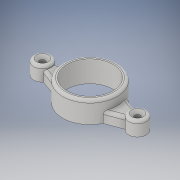
# Autodesk Inventor part: Counter_Support
Saved by Autodesk Inventor 2017 (Build 210142000, 142)
## iProperties
Created: 2019-12-30
Part Number: Counter_Support
Material: Generic
Document SubType Name: Modeling
Designer: Christian
Density: 1 g/cm^3
Appearance: Default
Author: Christian
Autodesk Inventor part; units mm, degrees
ref_plane "YZ Plane" through (0, 0, 0) normal (1, 0, 0) x (0, 1, 0)
ref_plane "XZ Plane" through (0, 0, 0) normal (0, 1, 0) x (-1, 0, 0)
ref_plane "XY Plane" through (0, 0, 0) normal (0, 0, 1) x (1, 0, 0)
sketch "Tube_Core_Skt" plane through (0, 0, 0) normal (0, 0, 1) x (1, 0, 0)
  circle A0 centre (0, 0) radius 16.025
  circle A1 centre (0, 0) radius 19.025
  dimension "d2" = 3
  dimension "d3" = 32.05
  constraints: 2 centre point, 2 coincident
  measures "d2" radial gap between concentric circles of A1 A0
  measures "d3" diameter of A0
extrude "Tube_Core" add sketch "Tube_Core_Skt" along normal blind 15
sketch "Screw_Core_Skt" plane through (0, 0, 0) normal (0, 1, 0) x (-1, 0, 0)
  line L0 (-19.025, 0) -> (-19.025, 15) projected
  line L1 (19.025, 15) -> (-19.025, 15) projected
  line L2 (19.025, 0) -> (19.025, 15) projected
  line L3 (-19.025, 0) -> (19.025, 0) projected
  line L4 (0, 15) -> (-27.025, 15) construction
  line L5 (-27.025, 15) -> (-27.025, 10) construction
  line L6 (-27.025, 0) -> (0, 0) construction
  line L7 (0, 0) -> (0, 15) construction
  line L8 (-27.025, 15) -> (-33.175, 15) construction
  line L9 (-33.175, 15) -> (-33.175, 0) construction
  line L10 (-33.175, 0) -> (-27.025, 0) construction
  line L11 (-33.175, 10) -> (-27.025, 10) construction
  line L12 (-27.025, 10) -> (-27.025, 0) construction
  line L13 (-31.175, 0) -> (-31.175, 7.85)
  line L14 (-31.175, 7.85) -> (-29.025, 10)
  line L15 (-27.025, 10) -> (-27.025, 0)
  line L16 (-31.175, 0) -> (-27.025, 0)
  line L17 (-29.025, 10) -> (-27.025, 10)
  point P0 (0, 0)
  dimension "d11" = 10
  dimension "d12" = 8
  dimension "d13" = 6.15
  dimension "d14" = 2
  dimension "d15" = 2
  dimension "d16" = 45
  constraints: 28 end point, 7 perpendicular, 4 collinear, 4 point on line, 3 parallel, 2 horizontal, 1 midpoint, 1 vertical
  measures "d11" distance between parallel lines of L10 L11
  measures "d12" distance between parallel lines of L0 L12
  measures "d13" distance between parallel lines of L9 L12
  measures "d14" distance between parallel lines of L9 L13
  measures "d15" distance of L14.end L5.end
  measures "d16" angle of L11 L14
revolve "Screw_Core" add sketch "Screw_Core_Skt" angle 360 about axis through (33.175, 0, 15) along (0, 0, -1) contours L13 L14 L17 L15 L16
sketch "Screw_Bridge_Skt" plane through (0, 0, 0) normal (0, 0, 1) x (1, 0, 0)
  circle A0 centre (0, 0) radius 19.025 projected
  circle A1 centre (33.175, 0) radius 6.15 projected
  circle A2 centre (0, 0) radius 19.025 projected
  line L0 (17.2095, 8.1107) -> (28.5035, 4)
  line L1 (17.2095, -8.1107) -> (28.5035, -4)
  line L2 (0, 0) -> (33.175, 0) construction
  point P0 (35.15, 0)
  dimension "d25" = 4
  dimension "d26" = 20
  constraints: 6 end point, 6 point on circle, 1 horizontal, 1 other
  measures "d25" distance from line of L2 L1.end
  measures "d26" angle of L2 L1
extrude "Screw_Bridge" add sketch "Screw_Bridge_Skt" along normal blind 7.5 contours A0 L0 A1 L1
mirror "Screw_Copy" about plane through (0, 0, 0) normal (1, 0, 0) of "Screw_Bridge", "Screw_Core"
fillet "Fillet" radius 2 7 edges at (-19.025, 0, 15) (22.8565, -6.0553, 7.5) (22.8565, 6.0553, 7.5) (39.325, 0, 10) (-22.8565, -6.0553, 7.5) (-22.8565, 6.0553, 7.5) (-39.325, 0, 10)
equation "\"d2\" = tube_wall_width"
equation "\"d3\" = tube_diam + tube_tolerance"
equation "\"d4\" = tube_wall_height"
equation "\"d11\" = screw_height"
equation "\"d12\" = screw_spacing"
equation "\"d13\" = 0.5 * screw_head_diam + screw_wall_width"
equation "\"d14\" = 0.5 * screw_tolerance + 0.5 * screw_body_diam"
equation "\"d15\" = screw_wall_width"
equation "\"d25\" = 2 * screw_wall_width"
equation "\"d27\" = 0.75 * screw_height"
equation "\"d41\" = fillet"
equation "\"tube_diam\" = 31.8"
equation "\"screw_body_diam\" = 3"
equation "\"screw_head_diam\" = 8.3"
equation "\"screw_head_height\" = 3"
equation "\"screw_spacing\" = 8"
equation "\"screw_height\" = 10"
equation "\"tube_tolerance\" = 0.25"
equation "\"tube_wall_width\" = 3"
equation "\"tube_wall_height\" = 15"
equation "\"screw_wall_width\" = 2"
equation "\"fillet\" = 2"
equation "\"tube_base\" = 2"
equation "\"tube_base_height\" = 2"
equation "\"screw_tolerance\" = 1"
equation "\"screw_length\" = 12.7"
equation "\"wood_width\" = 15"
equation "\"block_height\" = 15"
equation "\"screw_head_ang\" = 71.666667deg"
equation "\"screw_head_m\" = 71.666667deg"
body "Solid1"
